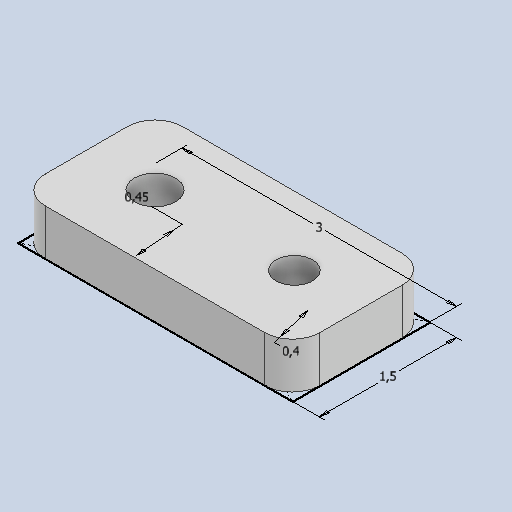
# Autodesk Inventor part: angulo
Saved by Autodesk Inventor 2024 (Build 280153000, 153)
## iProperties
Created: 2024-04-10
Part Number: angulo
Material: Generic
Document SubType Name: Modeling
Designer: JDAM
Density: 1 g/cm^3
Appearance: Default
Author: JDAM
Autodesk Inventor part; units mm, degrees
ref_plane "YZ Plane" through (0, 0, 0) normal (1, 0, 0) x (0, 1, 0)
ref_plane "XZ Plane" through (0, 0, 0) normal (0, 1, 0) x (-1, 0, 0)
ref_plane "XY Plane" through (0, 0, 0) normal (0, 0, 1) x (1, 0, 0)
sketch "Sketch1" plane through (0, 0, 0) normal (0, 1, 0) x (-1, 0, 0)
  line L0 (15, 7.5) -> (-15, 7.5)
  line L1 (-15, 7.5) -> (-15, -7.5)
  line L2 (-15, -7.5) -> (15, -7.5)
  line L3 (15, -7.5) -> (15, 7.5)
  line L4 (15, 7.5) -> (-15, -7.5) construction
  line L5 (-15, 7.5) -> (15, -7.5) construction
  line L6 (0, 7.5) -> (0, -7.5)
  line L7 (15, 0) -> (0, 0)
  circle A0 centre (7.5, 0) radius 2.25
  circle A1 centre (-7.7235, 0) radius 2
  dimension "d0" = 30
  dimension "d1" = 15
  dimension "d2" = 4.5
  dimension "d11" = 4
  constraints: 16 end point, 6 midpoint, 2 centre point, 2 horizontal, 2 parallel, 1 perpendicular
  measures "d0" distance of L2.end L1.end
  measures "d1" distance of L1.end L0.end
  measures "d2" diameter of A0
  measures "d11" diameter of A1
extrude "Extrusion1" add sketch "Sketch1" along normal blind 5 contours L3 L7 A0 L6 L0 | L6 L2 L1 L0 | L3 L2 L6 L7 A0
fillet "Fillet1" radius 3 4 edges at (-15, 2.5, 7.5) (-15, 2.5, -7.5) (15, 2.5, 7.5) (15, 2.5, -7.5)
body "Solid1"
